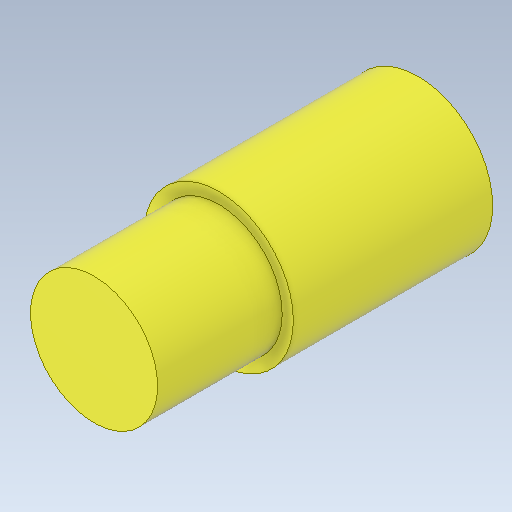
# Autodesk Inventor part: ピニオン　m0.5　10t
Saved by Autodesk Inventor 2020.2 (Build 242310000, 310)
## iProperties
Created: 2016-01-15
Part Number: ピニオン　m0.5　10t
Material: 一般
Document SubType Name: Modeling
Designer: Takumi
Density: 15.2283 g/cm^3
Appearance: 滑らか - 黄
Mass: 5 g
Surface Area: 2.87456 cm^2
Volume: 0.328336 cm^3
Author: Takumi
Autodesk Inventor part; units mm, degrees
ref_plane "YZ Plane" through (0, 0, 0) normal (1, 0, 0) x (0, 1, 0)
ref_plane "XZ Plane" through (0, 0, 0) normal (0, 1, 0) x (-1, 0, 0)
ref_plane "XY Plane" through (0, 0, 0) normal (0, 0, 1) x (1, 0, 0)
sketch "スケッチ1" plane through (0, 0, 0) normal (0, 0, 1) x (1, 0, 0)
  circle A0 centre (0, 0) radius 3
  circle A1 centre (0, 0) radius 2.55
  dimension "d0" = 6
  dimension "d1" = 5.1
  constraints: 2 centre point, 2 coincident
  measures "d0" diameter of A0
  measures "d1" diameter of A1
extrude "押し出し1" add sketch "スケッチ1" along normal blind 13 contours A1
extrude "押し出し2" add sketch "スケッチ1" along normal blind 8
